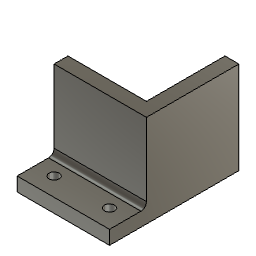
Laptop Mount FL_RR v1 (Autodesk Fusion 360 design; units mm, degrees)
Autodesk Fusion 360 part; units mm, degrees
sketch "Sketch1" plane through (0, 0, 0) normal (0, 0, 1) x (1, 0, 0)
  line L0 (0, 0) -> (50, 0)
  line L1 (50, 0) -> (50, 50)
  line L2 (0, 7.5) -> (42.5, 7.5)
  line L3 (42.5, 7.5) -> (42.5, 50)
  line L4 (0, 7.5) -> (0, 0)
  line L5 (42.5, 50) -> (50, 50)
  dimension "d1" = -7.5
  dimension "d2" = 50
  dimension "d3" = 50
  constraint coincident L0.start L4.end
  constraint horizontal L0
  constraint perpendicular L0 L1
  constraint perpendicular L2 L4
  constraint perpendicular L1 L5
  measures "d2" distance of L0.start L0.end
  measures "d3" distance of L0.end L1.end
extrude "Extrude1" add sketch "Sketch1" along normal blind 50
sketch "Sketch4" plane through (0, 0, 0) normal (0, 0, 1) x (1, 0, 0)
  line L0 (50, -20) -> (0, -20)
  line L1 (0, -20) -> (0, 50)
  line L2 (0, 50) -> (50, 50)
  line L3 (50, 50) -> (50, -20)
  point P0 (50, 50)
  dimension "d43" = 70
  dimension "d44" = 50
  constraint horizontal L0
  constraint vertical L1
  constraint horizontal L2
  constraint vertical L3
  constraint coincident P0 L2.end
  measures "d43" distance of L0.end L1.end
  measures "d44" distance of L1.end P0
extrude "Extrude4" add sketch "Sketch4" along normal blind 7.5
sketch "Sketch7" plane through (0, 0, 7.5) normal (0, 0, 1) x (-1, 0, 0)
  line L0 (0, 0) -> (0, 20)
  line L1 (-50, 0) -> (0, 0)
  line L2 (0, 20) -> (-50, 20)
  line L3 (-50, 20) -> (-50, 0)
  point P0 (-10, 10)
  point P1 (-40, 10)
  dimension "d35" = 30
  measures "d35" distance of P0 P1
hole "Hole1" at (10, -10, 7.5) at (40, -10, 7.5) direction (0, 0, -1) diameter 5.5 depth 10 tip angle 118
fillet "Fillet1" radius 3 1 edges at (25, 0, 7.5)
fillet "Fillet1" radius 3 2 edges at (21.25, 7.5, 7.5) (42.5, 28.75, 7.5)
